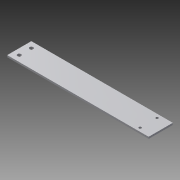
# Autodesk Inventor part: pre
Saved by Autodesk Inventor 2015 (Build 190159000, 159)
## iProperties
Created: 2015-06-22
Part Number: pre
Material: アルミニウム 5052 H32
Document SubType Name: Modeling
Designer: kenta
Density: 2.68 g/cm^3
Appearance: サテン
Author: kenta
Autodesk Inventor part; units mm, degrees
ref_plane "YZ Plane" through (0, 0, 0) normal (1, 0, 0) x (0, 1, 0)
ref_plane "XZ Plane" through (0, 0, 0) normal (0, 1, 0) x (-1, 0, 0)
ref_plane "XY Plane" through (0, 0, 0) normal (0, 0, 1) x (1, 0, 0)
sketch "スケッチ1" plane through (0, 0, 0) normal (0, 0, 1) x (1, 0, 0)
  line L0 (56, 10) -> (-56, 10)
  line L1 (-56, 10) -> (-56, -10)
  line L2 (-56, -10) -> (56, -10)
  line L3 (56, -10) -> (56, 10)
  line L4 (56, 10) -> (-56, -10) construction
  line L5 (-56, 10) -> (56, -10) construction
  point P0 (0, 0)
  dimension "d0" = 112
  dimension "d1" = 20
  constraints: 12 end point, 2 midpoint, 2 parallel, 1 horizontal, 1 perpendicular
  measures "d0" distance of L2.end L1.end
  measures "d1" distance of L1.end L0.end
extrude "押し出し1" add sketch "スケッチ1" along normal blind 1.5
sketch "スケッチ3" plane through (0, 0, 1.5) normal (0, 0, 1) x (1, 0, 0)
  line L0 (56, 10) -> (-56, 10) projected
  line L1 (-56, 10) -> (-56, -10) projected
  point P0 (0, 0)
  point P1 (-51, 5)
  point P2 (-51, -5)
  dimension "d10" = 10
  dimension "d11" = 5
  dimension "d12" = 5
  constraints: 1 vertical alignment
  measures "d10" distance of point (-51, -5) point (-51, 5)
  measures "d11" distance from line of point (-51, 5) L0
  measures "d12" distance from line of L1 point (-51, 5)
hole "穴1" at (-51, 5, 1.5) at (-51, -5, 1.5) direction (0, 0, -1) diameter 3 end through all
sketch "スケッチ5" plane through (0, 0, 1.5) normal (0, 0, 1) x (1, 0, 0)
  point P0 (0, 0)
  point P1 (51, 7)
  point P2 (51, -7)
hole "穴3" at (51, 7, 1.5) at (51, -7, 1.5) direction (0, 0, -1) diameter 2.1 end through all
sketch "スケッチ6" plane through (56, -10, 0) normal (1, 0, 0) x (0, 0, -1)
  line L0 (-1.5, 0) -> (0, 0)
  line L1 (0, 0) -> (0, 20)
  line L2 (0, 20) -> (-1.5, 20)
  line L3 (-1.5, 20) -> (-1.5, 0)
  point P0 (0, 10)
  dimension "d36" = 1.5
  dimension "d37" = 20
  constraints: 8 end point, 2 parallel, 1 horizontal, 1 perpendicular
  measures "d36" distance of L2.end L1.end
  measures "d37" distance of L1.end L0.end
extrude "押し出し3" add sketch "スケッチ6" along normal blind 5
